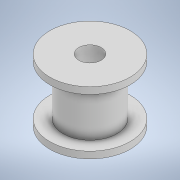
# Autodesk Inventor part: 5mm_bore_10mm_width_idlepulley
Saved by Autodesk Inventor 2021 (Build 250183000, 183)
## iProperties
Created: 2021-08-09
Part Number: 5mm_bore_10mm_width_idlepulley
Material: Generic
Document SubType Name: Modeling
Designer: Jorian Brusind
Density: 1 g/cm^3
Appearance: Default
Author: Jorian Brusind
Autodesk Inventor part; units mm, degrees
ref_plane "YZ Plane" through (0, 0, 0) normal (1, 0, 0) x (0, 1, 0)
ref_plane "XZ Plane" through (0, 0, 0) normal (0, 1, 0) x (-1, 0, 0)
ref_plane "XY Plane" through (0, 0, 0) normal (0, 0, 1) x (1, 0, 0)
sketch "Sketch1" plane through (0, 0, 0) normal (0, 1, 0) x (-1, 0, 0)
  circle A0 centre (0, 0) radius 9
  dimension "d0" = 18
  constraints: 1 centre point, 1 coincident
  measures "d0" diameter of A0
extrude "Extrusion1" add sketch "Sketch1" along normal blind 14
sketch "Sketch2" plane through (0, 14, 0) normal (0, 1, 0) x (1, 0, 0)
  circle A0 centre (0, 0) radius 2.5
  dimension "d3" = 5
  constraints: 1 centre point, 1 coincident
  measures "d3" diameter of A0
extrude "Extrusion2" cut sketch "Sketch2" against normal through all
sketch "Sketch3" plane through (0, 0, 0) normal (1, 0, 0) x (0, 1, 0)
  line L0 (0, 0) -> (14, 0)
  line L1 (14, -9) -> (14, 9) projected
  line L2 (7, 0) -> (7, -9)
  line L3 (0, -9) -> (14, -9) projected
  line L4 (1.5, -12) -> (12.5, -12)
  line L5 (12.5, -12) -> (12.5, -6)
  line L6 (12.5, -6) -> (1.5, -6)
  line L7 (1.5, -6) -> (1.5, -12)
  line L8 (1.5, -12) -> (12.5, -6) construction
  line L9 (12.5, -12) -> (1.5, -6) construction
  dimension "d6" = 14
  dimension "d7" = 11
  dimension "d8" = 6
  constraints: 16 end point, 5 midpoint, 2 parallel, 1 horizontal, 1 perpendicular
  measures "d6" distance of L0.start L0.end
  measures "d7" distance of L6.end L5.end
  measures "d8" distance of L5.end L4.end
revolve "Revolution1" cut sketch "Sketch3" angle 360 about axis through (0, 0, 0) along (0, 1, 0) contours L6 L5 L3 L2 | L2 L3 L7 L6 | L3 L5 L4 L7
body "Solid1"
